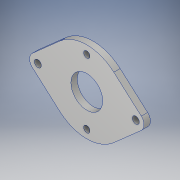
# Autodesk Inventor part: Motor Mount
Saved by Autodesk Inventor 2019.4 (Build 234330000, 330)
## iProperties
Created: 2020-01-27
Part Number: Motor Mount
Material: Aluminum 6061
Document SubType Name: Modeling
Designer: admin
Density: 2.7 g/cm^3
Appearance: Aluminum - Flat
Author: admin
Autodesk Inventor part; units mm, degrees
ref_plane "YZ Plane" through (0, 0, 0) normal (1, 0, 0) x (0, 1, 0)
ref_plane "XZ Plane" through (0, 0, 0) normal (0, 1, 0) x (-1, 0, 0)
ref_plane "XY Plane" through (0, 0, 0) normal (0, 0, 1) x (1, 0, 0)
sketch "Sketch1" plane through (0, 0, 0) normal (0, 0, 1) x (1, 0, 0)
  arc A0 (-21.1948, 23.9746) -> (-21.1948, -23.9746) centre (0, 0) ccw construction
  arc A1 (42.8052, 4.8698) -> (42.8052, -4.8698) centre (38.5, 0) ccw construction
  arc A2 (-42.8052, -4.8698) -> (-42.8052, 4.8698) centre (-38.5, 0) ccw construction
  circle A3 centre (-38.5, 0) radius 2.75
  circle A4 centre (38.5, 0) radius 2.75
  line L0 (38.5, 0) -> (-38.5, 0) construction
  line L1 (0, 25.4) -> (0, -25.4) construction
  circle A5 centre (0, 25.4) radius 2.5
  circle A6 centre (0, -25.4) radius 2.5
  line L2 (-42.8052, 4.8698) -> (-21.1948, 23.9746)
  line L3 (21.1948, 23.9746) -> (42.8052, 4.8698)
  line L4 (42.8052, -4.8698) -> (21.1948, -23.9746)
  line L5 (-42.8052, -4.8698) -> (-21.1948, -23.9746)
  arc A7 (-42.8052, 4.8698) -> (-42.8052, -4.8698) centre (-38.5, 0) ccw
  arc A8 (21.1948, 23.9746) -> (-21.1948, 23.9746) centre (0, 0) ccw
  arc A9 (21.1948, -23.9746) -> (21.1948, 23.9746) centre (0, 0) ccw construction
  arc A10 (42.8052, -4.8698) -> (42.8052, 4.8698) centre (38.5, 0) ccw
  arc A11 (-21.1948, -23.9746) -> (21.1948, -23.9746) centre (0, 0) ccw
  circle A12 centre (0, 0) radius 12.5
  dimension "d0" = 64
  dimension "d1" = 13
  dimension "d2" = 13
  dimension "d3" = 5.5
  dimension "d4" = 5.5
  dimension "d5" = 5
  dimension "d6" = 5
  dimension "d7" = 50.8
  dimension "d8" = 25
  constraints: 17 point on circle, 17 tangent, 13 centre point, 12 end point, 6 coincident, 3 midpoint, 1 horizontal, 1 vertical
  measures "d0" diameter of A0
  measures "d1" diameter of A1
  measures "d2" diameter of A2
  measures "d3" diameter of A3
  measures "d4" diameter of A4
  measures "d5" diameter of A5
  measures "d6" diameter of A6
  measures "d7" distance of L1.start L1.end
  measures "d8" diameter of A12
extrude "Extrusion1" add sketch "Sketch1" along normal blind 5
body "Solid1"
